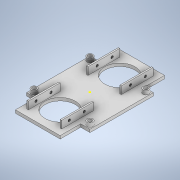
# Autodesk Inventor part: hydra_spider_v4_o
Saved by Autodesk Inventor 2020 (Build 240168000, 168)
## iProperties
Created: 2022-08-29
Part Number: hydra_spider_v4_o
Material: Generic
Document SubType Name: Modeling
Designer: Administrator
Density: 1 g/cm^3
Appearance: Default
Author: Administrator
Autodesk Inventor part; units mm, degrees
ref_plane "YZ Plane" through (0, 0, 0) normal (1, 0, 0) x (0, 1, 0)
ref_plane "XZ Plane" through (0, 0, 0) normal (0, 1, 0) x (-1, 0, 0)
ref_plane "XY Plane" through (0, 0, 0) normal (0, 0, 1) x (1, 0, 0)
sketch "Sketch1" plane through (0, 0, 0) normal (0, 1, 0) x (-1, 0, 0)
  line L0 (-42.5, -42.5) -> (42.5, -42.5)
  line L1 (42.5, -42.5) -> (42.5, 42.5)
  line L2 (42.5, 42.5) -> (-42.5, 42.5)
  line L3 (-42.5, 42.5) -> (-42.5, -42.5)
  line L4 (-45, -45) -> (40, 40) construction
  line L5 (40, -45) -> (-45, 40) construction
  line L6 (37.5, -37.5) -> (37.5, 37.5)
  line L7 (37.5, 37.5) -> (-37.5, 37.5)
  line L8 (-37.5, -37.5) -> (37.5, 37.5) construction
  line L9 (37.5, -37.5) -> (-37.5, 37.5) construction
  circle A0 centre (37.5, 37.5) radius 2.6
  line L10 (-36, -36) -> (36, 36) construction
  line L11 (36, -36) -> (-36, 36) construction
  circle A1 centre (37.5, -37.5) radius 2.6
  circle A2 centre (-37.5, 37.5) radius 2.6
  circle A3 centre (-37.5, -37.5) radius 2.6
  line L12 (30, -40) -> (-30, -40)
  line L13 (-30, -40) -> (-30, -70)
  line L14 (-30, -70) -> (30, -70)
  line L15 (30, -70) -> (30, -40)
  line L16 (-30, -40) -> (-30, 40)
  line L17 (30, 70) -> (-30, 70)
  line L18 (-30, 70) -> (-30, 40)
  line L19 (-30, 40) -> (30, 40)
  line L20 (30, 40) -> (30, 70)
  circle A4 centre (0, -40) radius 20.25
  circle A5 centre (0, 40) radius 20.25
  line L21 (55.4392, 43.942) -> (57.9392, 43.942)
  line L22 (57.9392, 43.942) -> (57.9392, 46.442)
  point P0 (20.0951, 37.5)
  point P1 (-20.0951, 37.5)
  point P2 (-30, 42.5)
  point P3 (-30, -42.5)
  point P4 (30, -42.5)
  point P5 (30, 42.5)
  point P6 (-20.0951, 42.5)
  point P7 (20.0951, 42.5)
  point P8 (37.5, 34.9)
  point P9 (34.9, 37.5)
  dimension "d0" = 85
  dimension "d1" = 85
  dimension "d2" = 75
  dimension "d3" = 75
  dimension "d4" = 5.2
  dimension "d5" = 72
  dimension "d6" = 72
  dimension "d9" = 75
  dimension "d12" = 75
  dimension "d164" = 60
  dimension "d165" = 30
  dimension "d170" = 60
  dimension "d171" = 30
  dimension "d172" = 40.5
  dimension "d173" = 40.5
  dimension "d441" = 2.5
  dimension "d442" = 2.5
  constraints: 46 end point, 6 centre point, 6 parallel, 5 horizontal, 5 perpendicular, 2 midpoint, 1 coincident, 1 vertical, 6 other
  measures "d0" distance of L2.end L1.end
  measures "d1" distance of L1.end L0.end
  measures "d2" distance of L7.end L6.end
  measures "d3" distance of L6.end L6.start
  measures "d4" diameter of A0
  measures "d5" distance of L11.end L10.end
  measures "d6" distance of L10.end L11.start
  measures "d9" distance of A0.centre A1.centre
  measures "d12" distance of A0.centre A2.centre
  measures "d164" distance of L14.end L13.end
  measures "d165" distance of L12.end L13.end
  measures "d170" distance of L20.start L18.end
  measures "d171" distance of L17.end L18.end
  measures "d172" diameter of A4
  measures "d173" diameter of A5
  measures "d441" distance of L21.start L21.end
  measures "d442" distance of L21.end L22.end
extrude "Extrusion1" add sketch "Sketch1" along normal blind 4 contours A2 | L3 L2 L18 L16 L13 L0 | L13 L12 A4 L0 | L0 A4 L15 L14 L13 | A1 | A0 L6 L7 | L7 L6 A0 | L16 L7 A5 L19 L20 L2 L1 L0 L15 L12 A4 | L18 L17 L20 L2 A5 | L2 A5 L19 L18 | A4 L12 L15 L0 | L16 L19 A5 L7 | L2 L20 L19 A5 | A3
sketch "Sketch2" plane through (0, 4, 0) normal (0, 1, 0) x (1, 0, 0)
  line L0 (0, 0) -> (21.3, 0)
  line L1 (21.3, 61.3) -> (21.3, 18.7)
  line L2 (21.3, 61.3) -> (-21.3, 61.3)
  line L3 (-21.3, 61.3) -> (-21.3, 18.7)
  line L4 (-21.3, 18.7) -> (-23.3, 18.7)
  line L5 (-23.3, 18.7) -> (-23.3, 61.3)
  line L6 (23.3, 61.3) -> (23.3, 18.7)
  line L7 (23.3, 18.7) -> (21.3, 18.7)
  line L8 (21.3, -61.3) -> (21.3, -18.7)
  line L9 (-21.3, -61.3) -> (-21.3, -18.7)
  line L10 (-21.3, -18.7) -> (-23.3, -18.7)
  line L11 (-23.3, -18.7) -> (-23.3, -61.3)
  line L12 (23.3, -61.3) -> (23.3, -18.7)
  line L13 (23.3, -18.7) -> (21.3, -18.7)
  line L14 (-23.3, -61.3) -> (-21.3, -61.3)
  line L15 (21.3, -61.3) -> (23.3, -61.3)
  line L16 (-23.3, 61.3) -> (-21.3, 61.3)
  line L17 (21.3, 61.3) -> (23.3, 61.3)
  line L18 (-23.3, 63.3) -> (-21.3, 63.3)
  line L19 (21.3, 63.3) -> (23.3, 63.3)
  dimension "d176" = 42.6
  dimension "d177" = 42.6
  dimension "d178" = 42.6
  dimension "d179" = 2
  dimension "d180" = 44.6
  dimension "d181" = 46.6
  constraints: 40 end point, 10 perpendicular, 6 symmetric about line, 5 point on line, 2 horizontal
  measures "d176" distance of L1.start L1.end
  measures "d177" distance of L1.start L2.end
  measures "d178" distance of L2.end L3.end
  measures "d179" distance of L3.end L4.end
  measures "d180" distance of L4.end L18.start
  measures "d181" distance of L18.start L19.end
extrude "Extrusion2" add sketch "Sketch2" along normal blind 10
sketch "Sketch18" plane through (-23.3, 4, 18.7) normal (-1, 0, 0) x (0, 0, 1)
  line L0 (-80, 10) -> (-37.4, 10) projected
  line L1 (-59.7, 10) -> (-59.7, 0)
  line L2 (-88.7, 0) -> (-61.2, 0) projected
  line L3 (-49.7, 5) -> (-69.7, 5)
  line L4 (42.6, 10) -> (0, 10) projected
  line L5 (22.3, 10) -> (22.3, 0)
  line L6 (51.3, 0) -> (23.8, 0) projected
  circle A0 centre (-49.7, 5) radius 1.65
  circle A1 centre (-69.7, 5) radius 1.65
  line L7 (-59.7, 0) -> (-59.7, 5)
  line L8 (22.3, 0) -> (22.3, 5)
  circle A2 centre (32.3, 5) radius 1.65
  circle A3 centre (12.3, 5) radius 1.65
  point P0 (-18.7, -4)
  point P1 (-82, 10)
  point P2 (44.6, 10)
  dimension "d191" = 20
  dimension "d192" = 3.3
  dimension "d193" = 3.3
  dimension "d194" = 20
  dimension "d195" = 3.3
  dimension "d196" = 3.3
  constraints: 10 end point, 4 centre point, 4 coincident, 4 point on line, 2 midpoint, 2 vertical
  measures "d191" distance of L3.start L3.end
  measures "d192" diameter of A0
  measures "d193" diameter of A1
  measures "d194" distance of point (32.3, 5) point (12.3, 5)
  measures "d195" diameter of A2
  measures "d196" diameter of A3
extrude "Extrusion6" cut sketch "Sketch18" against normal through all
thread "Thread7" size "M3x0.5" class "6H" standard "ANSI Metric M Profile" full length
thread "Thread8" size "M3x0.5" class "6H" standard "ANSI Metric M Profile" full length
thread "Thread11" size "M3x0.5" class "6H" standard "ANSI Metric M Profile" full length
thread "Thread12" size "M3x0.5" class "6H" standard "ANSI Metric M Profile" full length
thread "Thread13" size "M3x0.5" class "6H" standard "ANSI Metric M Profile" full length
thread "Thread14" size "M3x0.5" class "6H" standard "ANSI Metric M Profile" full length
thread "Thread15" size "M3x0.5" class "6H" standard "ANSI Metric M Profile" full length
thread "Thread16" size "M3x0.5" class "6H" standard "ANSI Metric M Profile" full length
sketch "Sketch20" plane through (-21.3, 9, -31) normal (0, -1, 0) x (0, 0, 1)
  line L0 (1.65, 0) -> (1.65, 2)
  line L1 (1.65, 2) -> (1.2793, 2)
  line L2 (1.2793, 2) -> (1.2793, 0)
  line L3 (1.2793, 0) -> (1.65, 0)
  line L4 (0, -25.96) -> (0, 6.66) projected
  constraints: 8 end point
revolve "Revolution7" add sketch "Sketch20" angle 360 about axis through (-21.3, 9, -31) along (-1, 0, 0) separate body
sketch "Sketch19" plane through (-21.3, 9, -29.35) normal (0, 1, 0) x (-1, 0, 0)
  line L0 (-0.2918, -0.0255) -> (-0.2501, -0.0255) construction
  line L1 (0.0416, -0.3456) -> (-0.0001, -0.4257) construction
  line L2 (-0.5001, -0.4257) -> (-0.5418, -0.3456) construction
  line L3 (-0.2084, -0.0255) -> (-0.2501, 0.0546) construction
  line L4 (-0.2501, 0.0546) -> (-0.2918, -0.0255) construction
  line L5 (-0.5001, -0.4257) -> (-0.4584, -0.3456) construction
  line L6 (-0.2084, -0.0255) -> (-0.0418, -0.3456)
  line L7 (-0.5418, -0.3456) -> (-0.4584, -0.3456) construction
  arc A0 (-0.5418, -0.3456) -> (-0.5001, -0.3709) centre (-0.5001, -0.3239) ccw construction
  line L8 (0.0416, -0.3456) -> (-0.0418, -0.3456) construction
  line L9 (-0.5001, -0.4257) -> (-0.5001, -0.3456) construction
  line L10 (-0.0001, -0.4257) -> (-0.0001, -0.3456) construction
  line L11 (-0.2501, 0.0546) -> (-0.2501, -0.0002) construction
  line L12 (-0.5001, -0.3709) -> (-0.0001, -0.3709)
  arc A1 (-0.5001, -0.3709) -> (-0.4584, -0.3456) centre (-0.5001, -0.3239) ccw
  line L13 (-0.0418, -0.3456) -> (-0.0001, -0.4257) construction
  line L14 (-0.4584, -0.3456) -> (-0.2918, -0.0255)
  line L15 (-0.0001, -0.0002) -> (-0.0001, 0.0177)
  line L16 (-0.0001, 0.0177) -> (-0.0001, -0.0002)
  line L17 (-0.0001, -0.0002) -> (0.0334, -0.0002)
  arc A2 (-0.0418, -0.3456) -> (-0.0001, -0.3709) centre (-0.0001, -0.3239) ccw
  arc A3 (-0.0001, -0.3709) -> (0.0416, -0.3456) centre (-0.0001, -0.3239) ccw construction
  arc A4 (-0.2501, -0.0002) -> (-0.2918, -0.0255) centre (-0.2501, -0.0471) ccw
  arc A5 (-0.2084, -0.0255) -> (-0.2501, -0.0002) centre (-0.2501, -0.0471) ccw
  line L18 (-0.2501, -0.0002) -> (-0.2501, -0.0255) construction
  line L19 (-0.2501, -0.0255) -> (-0.2084, -0.0255) construction
  dimension "d225" = 55
  dimension "d226" = 0.08
  dimension "d227" = 0.08
  dimension "Sketch19_ThreadOffset" = 0
  dimension "Sketch19_MajorRadius" = 0.3707
  dimension "d230" = 0.5
  dimension "Sketch19_MinorRadius" = 0
  constraints: 40 end point, 12 point on circle, 10 parallel, 8 tangent, 6 centre point, 6 collinear, 2 midpoint, 2 point on line, 1 horizontal, 1 perpendicular, 3 other
  measures "d225" angle of L6 L14
  measures "d226" distance of L3.end L0.end
  measures "d227" distance of L1.end L10.end
  measures "Sketch19_ThreadOffset" distance between parallel lines of L15 L10
  measures "Sketch19_MajorRadius" distance from line of L12 L15.start
  measures "d230" distance from line of L1.end L9
  measures "Sketch19_MinorRadius" distance edge to line of A5 L17
coil "Coil7" sketch "Sketch19" operation cut axis through (-21.3, 9, -31) along (-1, 0, 0) pitch 0.5005 turns 5.994006 hand right bodies 2
sketch "Sketch22" plane through (-21.3, 9, -51) normal (0, -1, 0) x (0, 0, 1)
  line L0 (1.65, 0) -> (1.65, 2)
  line L1 (1.65, 2) -> (1.2793, 2)
  line L2 (1.2793, 2) -> (1.2793, 0)
  line L3 (1.2793, 0) -> (1.65, 0)
  line L4 (0, -25.96) -> (0, 6.66) projected
  constraints: 8 end point
revolve "Revolution8" add sketch "Sketch22" angle 360 about axis through (-21.3, 9, -51) along (-1, 0, 0) separate body
sketch "Sketch21" plane through (-21.3, 9, -49.35) normal (0, 1, 0) x (-1, 0, 0)
  line L0 (-0.2918, -0.0255) -> (-0.2501, -0.0255) construction
  line L1 (0.0416, -0.3456) -> (-0.0001, -0.4257) construction
  line L2 (-0.5001, -0.4257) -> (-0.5418, -0.3456) construction
  line L3 (-0.2084, -0.0255) -> (-0.2501, 0.0546) construction
  line L4 (-0.2501, 0.0546) -> (-0.2918, -0.0255) construction
  line L5 (-0.5001, -0.4257) -> (-0.4584, -0.3456) construction
  line L6 (-0.2084, -0.0255) -> (-0.0418, -0.3456)
  line L7 (-0.5418, -0.3456) -> (-0.4584, -0.3456) construction
  arc A0 (-0.5418, -0.3456) -> (-0.5001, -0.3709) centre (-0.5001, -0.3239) ccw construction
  line L8 (0.0416, -0.3456) -> (-0.0418, -0.3456) construction
  line L9 (-0.5001, -0.4257) -> (-0.5001, -0.3456) construction
  line L10 (-0.0001, -0.4257) -> (-0.0001, -0.3456) construction
  line L11 (-0.2501, 0.0546) -> (-0.2501, -0.0002) construction
  line L12 (-0.5001, -0.3709) -> (-0.0001, -0.3709)
  arc A1 (-0.5001, -0.3709) -> (-0.4584, -0.3456) centre (-0.5001, -0.3239) ccw
  line L13 (-0.0418, -0.3456) -> (-0.0001, -0.4257) construction
  line L14 (-0.4584, -0.3456) -> (-0.2918, -0.0255)
  line L15 (-0.0001, -0.0002) -> (-0.0001, 0.0177)
  line L16 (-0.0001, 0.0177) -> (-0.0001, -0.0002)
  line L17 (-0.0001, -0.0002) -> (0.0334, -0.0002)
  arc A2 (-0.0418, -0.3456) -> (-0.0001, -0.3709) centre (-0.0001, -0.3239) ccw
  arc A3 (-0.0001, -0.3709) -> (0.0416, -0.3456) centre (-0.0001, -0.3239) ccw construction
  arc A4 (-0.2501, -0.0002) -> (-0.2918, -0.0255) centre (-0.2501, -0.0471) ccw
  arc A5 (-0.2084, -0.0255) -> (-0.2501, -0.0002) centre (-0.2501, -0.0471) ccw
  line L18 (-0.2501, -0.0002) -> (-0.2501, -0.0255) construction
  line L19 (-0.2501, -0.0255) -> (-0.2084, -0.0255) construction
  dimension "d243" = 55
  dimension "d244" = 0.08
  dimension "d245" = 0.08
  dimension "Sketch21_ThreadOffset" = 0
  dimension "Sketch21_MajorRadius" = 0.3707
  dimension "d248" = 0.5
  dimension "Sketch21_MinorRadius" = 0
  constraints: 40 end point, 12 point on circle, 10 parallel, 8 tangent, 6 centre point, 6 collinear, 2 midpoint, 2 point on line, 1 horizontal, 1 perpendicular, 3 other
  measures "d243" angle of L6 L14
  measures "d244" distance of L3.end L0.end
  measures "d245" distance of L1.end L10.end
  measures "Sketch21_ThreadOffset" distance between parallel lines of L15 L10
  measures "Sketch21_MajorRadius" distance from line of L12 L15.start
  measures "d248" distance from line of L1.end L9
  measures "Sketch21_MinorRadius" distance edge to line of A5 L17
coil "Coil8" sketch "Sketch21" operation cut axis through (-21.3, 9, -51) along (-1, 0, 0) pitch 0.5005 turns 5.994006 hand right bodies 3
sketch "Sketch28" plane through (23.3, 9, -51) normal (0, -1, 0) x (0, 0, 1)
  line L0 (1.65, 0) -> (1.65, 2)
  line L1 (1.65, 2) -> (1.2793, 2)
  line L2 (1.2793, 2) -> (1.2793, 0)
  line L3 (1.2793, 0) -> (1.65, 0)
  line L4 (0, -4.66) -> (0, 27.96) projected
  constraints: 8 end point
revolve "Revolution11" add sketch "Sketch28" angle 360 about axis through (23.3, 9, -51) along (-1, 0, 0) separate body
sketch "Sketch27" plane through (23.3, 9, -49.35) normal (0, 1, 0) x (-1, 0, 0)
  line L0 (-0.2918, -0.0255) -> (-0.2501, -0.0255) construction
  line L1 (0.0416, -0.3456) -> (-0.0001, -0.4257) construction
  line L2 (-0.5001, -0.4257) -> (-0.5418, -0.3456) construction
  line L3 (-0.2084, -0.0255) -> (-0.2501, 0.0546) construction
  line L4 (-0.2501, 0.0546) -> (-0.2918, -0.0255) construction
  line L5 (-0.5001, -0.4257) -> (-0.4584, -0.3456) construction
  line L6 (-0.2084, -0.0255) -> (-0.0418, -0.3456)
  line L7 (-0.5418, -0.3456) -> (-0.4584, -0.3456) construction
  arc A0 (-0.5418, -0.3456) -> (-0.5001, -0.3709) centre (-0.5001, -0.3239) ccw construction
  line L8 (0.0416, -0.3456) -> (-0.0418, -0.3456) construction
  line L9 (-0.5001, -0.4257) -> (-0.5001, -0.3456) construction
  line L10 (-0.0001, -0.4257) -> (-0.0001, -0.3456) construction
  line L11 (-0.2501, 0.0546) -> (-0.2501, -0.0002) construction
  line L12 (-0.5001, -0.3709) -> (-0.0001, -0.3709)
  arc A1 (-0.5001, -0.3709) -> (-0.4584, -0.3456) centre (-0.5001, -0.3239) ccw
  line L13 (-0.0418, -0.3456) -> (-0.0001, -0.4257) construction
  line L14 (-0.4584, -0.3456) -> (-0.2918, -0.0255)
  line L15 (-0.0001, -0.0002) -> (-0.0001, 0.0177)
  line L16 (-0.0001, 0.0177) -> (-0.0001, -0.0002)
  line L17 (-0.0001, -0.0002) -> (0.0334, -0.0002)
  arc A2 (-0.0418, -0.3456) -> (-0.0001, -0.3709) centre (-0.0001, -0.3239) ccw
  arc A3 (-0.0001, -0.3709) -> (0.0416, -0.3456) centre (-0.0001, -0.3239) ccw construction
  arc A4 (-0.2501, -0.0002) -> (-0.2918, -0.0255) centre (-0.2501, -0.0471) ccw
  arc A5 (-0.2084, -0.0255) -> (-0.2501, -0.0002) centre (-0.2501, -0.0471) ccw
  line L18 (-0.2501, -0.0002) -> (-0.2501, -0.0255) construction
  line L19 (-0.2501, -0.0255) -> (-0.2084, -0.0255) construction
  dimension "d297" = 55
  dimension "d298" = 0.08
  dimension "d299" = 0.08
  dimension "Sketch27_ThreadOffset" = 0
  dimension "Sketch27_MajorRadius" = 0.3707
  dimension "d302" = 0.5
  dimension "Sketch27_MinorRadius" = 0
  constraints: 40 end point, 12 point on circle, 10 parallel, 8 tangent, 6 centre point, 6 collinear, 2 midpoint, 2 point on line, 1 horizontal, 1 perpendicular, 3 other
  measures "d297" angle of L6 L14
  measures "d298" distance of L3.end L0.end
  measures "d299" distance of L1.end L10.end
  measures "Sketch27_ThreadOffset" distance between parallel lines of L15 L10
  measures "Sketch27_MajorRadius" distance from line of L12 L15.start
  measures "d302" distance from line of L1.end L9
  measures "Sketch27_MinorRadius" distance edge to line of A5 L17
coil "Coil11" sketch "Sketch27" operation cut axis through (23.3, 9, -51) along (-1, 0, 0) pitch 0.5005 turns 5.994006 hand right bodies 4
sketch "Sketch30" plane through (23.3, 9, -31) normal (0, -1, 0) x (0, 0, 1)
  line L0 (1.65, 0) -> (1.65, 2)
  line L1 (1.65, 2) -> (1.2793, 2)
  line L2 (1.2793, 2) -> (1.2793, 0)
  line L3 (1.2793, 0) -> (1.65, 0)
  line L4 (0, -4.66) -> (0, 27.96) projected
  constraints: 8 end point
revolve "Revolution12" add sketch "Sketch30" angle 360 about axis through (23.3, 9, -31) along (-1, 0, 0) separate body
sketch "Sketch29" plane through (23.3, 9, -29.35) normal (0, 1, 0) x (-1, 0, 0)
  line L0 (-0.2918, -0.0255) -> (-0.2501, -0.0255) construction
  line L1 (0.0416, -0.3456) -> (-0.0001, -0.4257) construction
  line L2 (-0.5001, -0.4257) -> (-0.5418, -0.3456) construction
  line L3 (-0.2084, -0.0255) -> (-0.2501, 0.0546) construction
  line L4 (-0.2501, 0.0546) -> (-0.2918, -0.0255) construction
  line L5 (-0.5001, -0.4257) -> (-0.4584, -0.3456) construction
  line L6 (-0.2084, -0.0255) -> (-0.0418, -0.3456)
  line L7 (-0.5418, -0.3456) -> (-0.4584, -0.3456) construction
  arc A0 (-0.5418, -0.3456) -> (-0.5001, -0.3709) centre (-0.5001, -0.3239) ccw construction
  line L8 (0.0416, -0.3456) -> (-0.0418, -0.3456) construction
  line L9 (-0.5001, -0.4257) -> (-0.5001, -0.3456) construction
  line L10 (-0.0001, -0.4257) -> (-0.0001, -0.3456) construction
  line L11 (-0.2501, 0.0546) -> (-0.2501, -0.0002) construction
  line L12 (-0.5001, -0.3709) -> (-0.0001, -0.3709)
  arc A1 (-0.5001, -0.3709) -> (-0.4584, -0.3456) centre (-0.5001, -0.3239) ccw
  line L13 (-0.0418, -0.3456) -> (-0.0001, -0.4257) construction
  line L14 (-0.4584, -0.3456) -> (-0.2918, -0.0255)
  line L15 (-0.0001, -0.0002) -> (-0.0001, 0.0177)
  line L16 (-0.0001, 0.0177) -> (-0.0001, -0.0002)
  line L17 (-0.0001, -0.0002) -> (0.0334, -0.0002)
  arc A2 (-0.0418, -0.3456) -> (-0.0001, -0.3709) centre (-0.0001, -0.3239) ccw
  arc A3 (-0.0001, -0.3709) -> (0.0416, -0.3456) centre (-0.0001, -0.3239) ccw construction
  arc A4 (-0.2501, -0.0002) -> (-0.2918, -0.0255) centre (-0.2501, -0.0471) ccw
  arc A5 (-0.2084, -0.0255) -> (-0.2501, -0.0002) centre (-0.2501, -0.0471) ccw
  line L18 (-0.2501, -0.0002) -> (-0.2501, -0.0255) construction
  line L19 (-0.2501, -0.0255) -> (-0.2084, -0.0255) construction
  dimension "d315" = 55
  dimension "d316" = 0.08
  dimension "d317" = 0.08
  dimension "Sketch29_ThreadOffset" = 0
  dimension "Sketch29_MajorRadius" = 0.3707
  dimension "d320" = 0.5
  dimension "Sketch29_MinorRadius" = 0
  constraints: 40 end point, 12 point on circle, 10 parallel, 8 tangent, 6 centre point, 6 collinear, 2 midpoint, 2 point on line, 1 horizontal, 1 perpendicular, 3 other
  measures "d315" angle of L6 L14
  measures "d316" distance of L3.end L0.end
  measures "d317" distance of L1.end L10.end
  measures "Sketch29_ThreadOffset" distance between parallel lines of L15 L10
  measures "Sketch29_MajorRadius" distance from line of L12 L15.start
  measures "d320" distance from line of L1.end L9
  measures "Sketch29_MinorRadius" distance edge to line of A5 L17
coil "Coil12" sketch "Sketch29" operation cut axis through (23.3, 9, -31) along (-1, 0, 0) pitch 0.5005 turns 5.994006 hand right bodies 5
sketch "Sketch32" plane through (23.3, 9, 31) normal (0, -1, 0) x (0, 0, 1)
  line L0 (1.65, 0) -> (1.65, 2)
  line L1 (1.65, 2) -> (1.2793, 2)
  line L2 (1.2793, 2) -> (1.2793, 0)
  line L3 (1.2793, 0) -> (1.65, 0)
  line L4 (0, -4.66) -> (0, 27.96) projected
  constraints: 8 end point
revolve "Revolution13" add sketch "Sketch32" angle 360 about axis through (23.3, 9, 31) along (-1, 0, 0) separate body
sketch "Sketch31" plane through (23.3, 9, 32.65) normal (0, 1, 0) x (-1, 0, 0)
  line L0 (-0.2918, -0.0255) -> (-0.2501, -0.0255) construction
  line L1 (0.0416, -0.3456) -> (-0.0001, -0.4257) construction
  line L2 (-0.5001, -0.4257) -> (-0.5418, -0.3456) construction
  line L3 (-0.2084, -0.0255) -> (-0.2501, 0.0546) construction
  line L4 (-0.2501, 0.0546) -> (-0.2918, -0.0255) construction
  line L5 (-0.5001, -0.4257) -> (-0.4584, -0.3456) construction
  line L6 (-0.2084, -0.0255) -> (-0.0418, -0.3456)
  line L7 (-0.5418, -0.3456) -> (-0.4584, -0.3456) construction
  arc A0 (-0.5418, -0.3456) -> (-0.5001, -0.3709) centre (-0.5001, -0.3239) ccw construction
  line L8 (0.0416, -0.3456) -> (-0.0418, -0.3456) construction
  line L9 (-0.5001, -0.4257) -> (-0.5001, -0.3456) construction
  line L10 (-0.0001, -0.4257) -> (-0.0001, -0.3456) construction
  line L11 (-0.2501, 0.0546) -> (-0.2501, -0.0002) construction
  line L12 (-0.5001, -0.3709) -> (-0.0001, -0.3709)
  arc A1 (-0.5001, -0.3709) -> (-0.4584, -0.3456) centre (-0.5001, -0.3239) ccw
  line L13 (-0.0418, -0.3456) -> (-0.0001, -0.4257) construction
  line L14 (-0.4584, -0.3456) -> (-0.2918, -0.0255)
  line L15 (-0.0001, -0.0002) -> (-0.0001, 0.0177)
  line L16 (-0.0001, 0.0177) -> (-0.0001, -0.0002)
  line L17 (-0.0001, -0.0002) -> (0.0334, -0.0002)
  arc A2 (-0.0418, -0.3456) -> (-0.0001, -0.3709) centre (-0.0001, -0.3239) ccw
  arc A3 (-0.0001, -0.3709) -> (0.0416, -0.3456) centre (-0.0001, -0.3239) ccw construction
  arc A4 (-0.2501, -0.0002) -> (-0.2918, -0.0255) centre (-0.2501, -0.0471) ccw
  arc A5 (-0.2084, -0.0255) -> (-0.2501, -0.0002) centre (-0.2501, -0.0471) ccw
  line L18 (-0.2501, -0.0002) -> (-0.2501, -0.0255) construction
  line L19 (-0.2501, -0.0255) -> (-0.2084, -0.0255) construction
  dimension "d333" = 55
  dimension "d334" = 0.08
  dimension "d335" = 0.08
  dimension "Sketch31_ThreadOffset" = 0
  dimension "Sketch31_MajorRadius" = 0.3707
  dimension "d338" = 0.5
  dimension "Sketch31_MinorRadius" = 0
  constraints: 40 end point, 12 point on circle, 10 parallel, 8 tangent, 6 centre point, 6 collinear, 2 midpoint, 2 point on line, 1 horizontal, 1 perpendicular, 3 other
  measures "d333" angle of L6 L14
  measures "d334" distance of L3.end L0.end
  measures "d335" distance of L1.end L10.end
  measures "Sketch31_ThreadOffset" distance between parallel lines of L15 L10
  measures "Sketch31_MajorRadius" distance from line of L12 L15.start
  measures "d338" distance from line of L1.end L9
  measures "Sketch31_MinorRadius" distance edge to line of A5 L17
coil "Coil13" sketch "Sketch31" operation cut axis through (23.3, 9, 31) along (-1, 0, 0) pitch 0.5005 turns 5.994006 hand right bodies 6
sketch "Sketch34" plane through (23.3, 9, 51) normal (0, -1, 0) x (0, 0, 1)
  line L0 (1.65, 0) -> (1.65, 2)
  line L1 (1.65, 2) -> (1.2793, 2)
  line L2 (1.2793, 2) -> (1.2793, 0)
  line L3 (1.2793, 0) -> (1.65, 0)
  line L4 (0, -4.66) -> (0, 27.96) projected
  constraints: 8 end point
revolve "Revolution14" add sketch "Sketch34" angle 360 about axis through (23.3, 9, 51) along (-1, 0, 0) separate body
sketch "Sketch33" plane through (23.3, 9, 52.65) normal (0, 1, 0) x (-1, 0, 0)
  line L0 (-0.2918, -0.0255) -> (-0.2501, -0.0255) construction
  line L1 (0.0416, -0.3456) -> (-0.0001, -0.4257) construction
  line L2 (-0.5001, -0.4257) -> (-0.5418, -0.3456) construction
  line L3 (-0.2084, -0.0255) -> (-0.2501, 0.0546) construction
  line L4 (-0.2501, 0.0546) -> (-0.2918, -0.0255) construction
  line L5 (-0.5001, -0.4257) -> (-0.4584, -0.3456) construction
  line L6 (-0.2084, -0.0255) -> (-0.0418, -0.3456)
  line L7 (-0.5418, -0.3456) -> (-0.4584, -0.3456) construction
  arc A0 (-0.5418, -0.3456) -> (-0.5001, -0.3709) centre (-0.5001, -0.3239) ccw construction
  line L8 (0.0416, -0.3456) -> (-0.0418, -0.3456) construction
  line L9 (-0.5001, -0.4257) -> (-0.5001, -0.3456) construction
  line L10 (-0.0001, -0.4257) -> (-0.0001, -0.3456) construction
  line L11 (-0.2501, 0.0546) -> (-0.2501, -0.0002) construction
  line L12 (-0.5001, -0.3709) -> (-0.0001, -0.3709)
  arc A1 (-0.5001, -0.3709) -> (-0.4584, -0.3456) centre (-0.5001, -0.3239) ccw
  line L13 (-0.0418, -0.3456) -> (-0.0001, -0.4257) construction
  line L14 (-0.4584, -0.3456) -> (-0.2918, -0.0255)
  line L15 (-0.0001, -0.0002) -> (-0.0001, 0.0177)
  line L16 (-0.0001, 0.0177) -> (-0.0001, -0.0002)
  line L17 (-0.0001, -0.0002) -> (0.0334, -0.0002)
  arc A2 (-0.0418, -0.3456) -> (-0.0001, -0.3709) centre (-0.0001, -0.3239) ccw
  arc A3 (-0.0001, -0.3709) -> (0.0416, -0.3456) centre (-0.0001, -0.3239) ccw construction
  arc A4 (-0.2501, -0.0002) -> (-0.2918, -0.0255) centre (-0.2501, -0.0471) ccw
  arc A5 (-0.2084, -0.0255) -> (-0.2501, -0.0002) centre (-0.2501, -0.0471) ccw
  line L18 (-0.2501, -0.0002) -> (-0.2501, -0.0255) construction
  line L19 (-0.2501, -0.0255) -> (-0.2084, -0.0255) construction
  dimension "d351" = 55
  dimension "d352" = 0.08
  dimension "d353" = 0.08
  dimension "Sketch33_ThreadOffset" = 0
  dimension "Sketch33_MajorRadius" = 0.3707
  dimension "d356" = 0.5
  dimension "Sketch33_MinorRadius" = 0
  constraints: 40 end point, 12 point on circle, 10 parallel, 8 tangent, 6 centre point, 6 collinear, 2 midpoint, 2 point on line, 1 horizontal, 1 perpendicular, 3 other
  measures "d351" angle of L6 L14
  measures "d352" distance of L3.end L0.end
  measures "d353" distance of L1.end L10.end
  measures "Sketch33_ThreadOffset" distance between parallel lines of L15 L10
  measures "Sketch33_MajorRadius" distance from line of L12 L15.start
  measures "d356" distance from line of L1.end L9
  measures "Sketch33_MinorRadius" distance edge to line of A5 L17
coil "Coil14" sketch "Sketch33" operation cut axis through (23.3, 9, 51) along (-1, 0, 0) pitch 0.5005 turns 5.994006 hand right bodies 7
sketch "Sketch36" plane through (-21.3, 9, 31) normal (0, -1, 0) x (0, 0, 1)
  line L0 (1.65, 0) -> (1.65, 2)
  line L1 (1.65, 2) -> (1.2793, 2)
  line L2 (1.2793, 2) -> (1.2793, 0)
  line L3 (1.2793, 0) -> (1.65, 0)
  line L4 (0, -25.96) -> (0, 6.66) projected
  constraints: 8 end point
revolve "Revolution15" add sketch "Sketch36" angle 360 about axis through (-21.3, 9, 31) along (-1, 0, 0) separate body
sketch "Sketch35" plane through (-21.3, 9, 32.65) normal (0, 1, 0) x (-1, 0, 0)
  line L0 (-0.2918, -0.0255) -> (-0.2501, -0.0255) construction
  line L1 (0.0416, -0.3456) -> (-0.0001, -0.4257) construction
  line L2 (-0.5001, -0.4257) -> (-0.5418, -0.3456) construction
  line L3 (-0.2084, -0.0255) -> (-0.2501, 0.0546) construction
  line L4 (-0.2501, 0.0546) -> (-0.2918, -0.0255) construction
  line L5 (-0.5001, -0.4257) -> (-0.4584, -0.3456) construction
  line L6 (-0.2084, -0.0255) -> (-0.0418, -0.3456)
  line L7 (-0.5418, -0.3456) -> (-0.4584, -0.3456) construction
  arc A0 (-0.5418, -0.3456) -> (-0.5001, -0.3709) centre (-0.5001, -0.3239) ccw construction
  line L8 (0.0416, -0.3456) -> (-0.0418, -0.3456) construction
  line L9 (-0.5001, -0.4257) -> (-0.5001, -0.3456) construction
  line L10 (-0.0001, -0.4257) -> (-0.0001, -0.3456) construction
  line L11 (-0.2501, 0.0546) -> (-0.2501, -0.0002) construction
  line L12 (-0.5001, -0.3709) -> (-0.0001, -0.3709)
  arc A1 (-0.5001, -0.3709) -> (-0.4584, -0.3456) centre (-0.5001, -0.3239) ccw
  line L13 (-0.0418, -0.3456) -> (-0.0001, -0.4257) construction
  line L14 (-0.4584, -0.3456) -> (-0.2918, -0.0255)
  line L15 (-0.0001, -0.0002) -> (-0.0001, 0.0177)
  line L16 (-0.0001, 0.0177) -> (-0.0001, -0.0002)
  line L17 (-0.0001, -0.0002) -> (0.0334, -0.0002)
  arc A2 (-0.0418, -0.3456) -> (-0.0001, -0.3709) centre (-0.0001, -0.3239) ccw
  arc A3 (-0.0001, -0.3709) -> (0.0416, -0.3456) centre (-0.0001, -0.3239) ccw construction
  arc A4 (-0.2501, -0.0002) -> (-0.2918, -0.0255) centre (-0.2501, -0.0471) ccw
  arc A5 (-0.2084, -0.0255) -> (-0.2501, -0.0002) centre (-0.2501, -0.0471) ccw
  line L18 (-0.2501, -0.0002) -> (-0.2501, -0.0255) construction
  line L19 (-0.2501, -0.0255) -> (-0.2084, -0.0255) construction
  dimension "d369" = 55
  dimension "d370" = 0.08
  dimension "d371" = 0.08
  dimension "Sketch35_ThreadOffset" = 0
  dimension "Sketch35_MajorRadius" = 0.3707
  dimension "d374" = 0.5
  dimension "Sketch35_MinorRadius" = 0
  constraints: 40 end point, 12 point on circle, 10 parallel, 8 tangent, 6 centre point, 6 collinear, 2 midpoint, 2 point on line, 1 horizontal, 1 perpendicular, 3 other
  measures "d369" angle of L6 L14
  measures "d370" distance of L3.end L0.end
  measures "d371" distance of L1.end L10.end
  measures "Sketch35_ThreadOffset" distance between parallel lines of L15 L10
  measures "Sketch35_MajorRadius" distance from line of L12 L15.start
  measures "d374" distance from line of L1.end L9
  measures "Sketch35_MinorRadius" distance edge to line of A5 L17
coil "Coil15" sketch "Sketch35" operation cut axis through (-21.3, 9, 31) along (-1, 0, 0) pitch 0.5005 turns 5.994006 hand right bodies 8
sketch "Sketch38" plane through (-21.3, 9, 51) normal (0, -1, 0) x (0, 0, 1)
  line L0 (1.65, 0) -> (1.65, 2)
  line L1 (1.65, 2) -> (1.2793, 2)
  line L2 (1.2793, 2) -> (1.2793, 0)
  line L3 (1.2793, 0) -> (1.65, 0)
  line L4 (0, -25.96) -> (0, 6.66) projected
  constraints: 8 end point
revolve "Revolution16" add sketch "Sketch38" angle 360 about axis through (-21.3, 9, 51) along (-1, 0, 0) separate body
sketch "Sketch37" plane through (-21.3, 9, 52.65) normal (0, 1, 0) x (-1, 0, 0)
  line L0 (-0.2918, -0.0255) -> (-0.2501, -0.0255) construction
  line L1 (0.0416, -0.3456) -> (-0.0001, -0.4257) construction
  line L2 (-0.5001, -0.4257) -> (-0.5418, -0.3456) construction
  line L3 (-0.2084, -0.0255) -> (-0.2501, 0.0546) construction
  line L4 (-0.2501, 0.0546) -> (-0.2918, -0.0255) construction
  line L5 (-0.5001, -0.4257) -> (-0.4584, -0.3456) construction
  line L6 (-0.2084, -0.0255) -> (-0.0418, -0.3456)
  line L7 (-0.5418, -0.3456) -> (-0.4584, -0.3456) construction
  arc A0 (-0.5418, -0.3456) -> (-0.5001, -0.3709) centre (-0.5001, -0.3239) ccw construction
  line L8 (0.0416, -0.3456) -> (-0.0418, -0.3456) construction
  line L9 (-0.5001, -0.4257) -> (-0.5001, -0.3456) construction
  line L10 (-0.0001, -0.4257) -> (-0.0001, -0.3456) construction
  line L11 (-0.2501, 0.0546) -> (-0.2501, -0.0002) construction
  line L12 (-0.5001, -0.3709) -> (-0.0001, -0.3709)
  arc A1 (-0.5001, -0.3709) -> (-0.4584, -0.3456) centre (-0.5001, -0.3239) ccw
  line L13 (-0.0418, -0.3456) -> (-0.0001, -0.4257) construction
  line L14 (-0.4584, -0.3456) -> (-0.2918, -0.0255)
  line L15 (-0.0001, -0.0002) -> (-0.0001, 0.0177)
  line L16 (-0.0001, 0.0177) -> (-0.0001, -0.0002)
  line L17 (-0.0001, -0.0002) -> (0.0334, -0.0002)
  arc A2 (-0.0418, -0.3456) -> (-0.0001, -0.3709) centre (-0.0001, -0.3239) ccw
  arc A3 (-0.0001, -0.3709) -> (0.0416, -0.3456) centre (-0.0001, -0.3239) ccw construction
  arc A4 (-0.2501, -0.0002) -> (-0.2918, -0.0255) centre (-0.2501, -0.0471) ccw
  arc A5 (-0.2084, -0.0255) -> (-0.2501, -0.0002) centre (-0.2501, -0.0471) ccw
  line L18 (-0.2501, -0.0002) -> (-0.2501, -0.0255) construction
  line L19 (-0.2501, -0.0255) -> (-0.2084, -0.0255) construction
  dimension "d387" = 55
  dimension "d388" = 0.08
  dimension "d389" = 0.08
  dimension "Sketch37_ThreadOffset" = 0
  dimension "Sketch37_MajorRadius" = 0.3707
  dimension "d392" = 0.5
  dimension "Sketch37_MinorRadius" = 0
  constraints: 40 end point, 12 point on circle, 10 parallel, 8 tangent, 6 centre point, 6 collinear, 2 midpoint, 2 point on line, 1 horizontal, 1 perpendicular, 3 other
  measures "d387" angle of L6 L14
  measures "d388" distance of L3.end L0.end
  measures "d389" distance of L1.end L10.end
  measures "Sketch37_ThreadOffset" distance between parallel lines of L15 L10
  measures "Sketch37_MajorRadius" distance from line of L12 L15.start
  measures "d392" distance from line of L1.end L9
  measures "Sketch37_MinorRadius" distance edge to line of A5 L17
coil "Coil16" sketch "Sketch37" operation cut axis through (-21.3, 9, 51) along (-1, 0, 0) pitch 0.5005 turns 5.994006 hand right bodies 9
sketch "Sketch43" plane through (0, 4, 0) normal (0, 1, 0) x (1, 0, 0)
  point P0 (0, 0)
sketch "Sketch44" plane through (0, 4, 0) normal (0, 1, 0) x (1, 0, 0)
  point P0 (0, 0)
sketch "Sketch45" plane through (0, 4, 0) normal (0, 1, 0) x (1, 0, 0)
  line L0 (37.5, 37.5) -> (-37.5, 37.5)
  line L1 (-37.5, 37.5) -> (-37.5, -37.5)
  line L2 (-37.5, -37.5) -> (37.5, -37.5)
  line L3 (37.5, -37.5) -> (37.5, 37.5)
  line L4 (37.5, 37.5) -> (-37.5, -37.5) construction
  line L5 (-37.5, 37.5) -> (37.5, -37.5) construction
  circle A0 centre (37.5, -37.5) radius 2.6
  circle A1 centre (-37.5, -37.5) radius 2.6
  circle A2 centre (37.5, 37.5) radius 2.6
  circle A3 centre (-37.5, 37.5) radius 2.6
  point P0 (0, 0)
  dimension "d443" = 75
  dimension "d444" = 75
  dimension "d445" = 5.2
  dimension "d448" = 75
  dimension "d451" = 75
  constraints: 12 end point, 4 centre point, 2 horizontal, 2 midpoint, 2 parallel, 1 coincident, 1 perpendicular, 1 vertical, 6 other
  measures "d443" distance of L2.end L1.end
  measures "d444" distance of L1.end L0.end
  measures "d445" diameter of A0
  measures "d448" distance of A0.centre A1.centre
  measures "d451" distance of A0.centre A2.centre
extrude "Extrusion7" cut sketch "Sketch45" against normal blind 2 contours A3 L1 L0 | L0 L1 A3 | A2 L3 L0 | L0 L3 A2 | A1 L2 L1 | L1 L2 A1 | A0 L2 L3 | L3 L2 A0 bodies 1
sketch "Sketch46" plane through (0, 4, 0) normal (0, 1, 0) x (1, 0, 0)
  circle A0 centre (37.5, -37.5) radius 2.6 projected
  circle A1 centre (37.5, -37.5) radius 2.6
  circle A2 centre (37.5, -37.5) radius 4
  line L0 (37.5, 37.5) -> (-37.5, 37.5)
  line L1 (-37.5, 37.5) -> (-37.5, -37.5)
  line L2 (-37.5, -37.5) -> (37.5, -37.5)
  line L3 (37.5, -37.5) -> (37.5, 37.5)
  line L4 (37.5, 37.5) -> (-37.5, -37.5) construction
  line L5 (-37.5, 37.5) -> (37.5, -37.5) construction
  circle A3 centre (-37.5, -37.5) radius 2.6
  circle A4 centre (-37.5, -37.5) radius 4
  circle A5 centre (37.5, 37.5) radius 2.6
  circle A6 centre (37.5, 37.5) radius 4
  circle A7 centre (-37.5, 37.5) radius 2.6
  circle A8 centre (-37.5, 37.5) radius 4
  point P0 (0, 0)
  dimension "d456" = 8
  dimension "d457" = 75
  dimension "d458" = 75
  dimension "d461" = 75
  dimension "d464" = 75
  constraints: 12 end point, 8 centre point, 8 coincident, 2 horizontal, 2 midpoint, 2 parallel, 1 perpendicular, 1 vertical, 18 other
  measures "d456" diameter of A2
  measures "d457" distance of L2.end L1.end
  measures "d458" distance of L1.end L0.end
  measures "d461" distance of A1.centre A3.centre
  measures "d464" distance of A1.centre A5.centre
extrude "Extrusion8" add sketch "Sketch46" along normal blind 5 contours A0 L3 A2 L2 | A0 L2 A2 L3 | A6 L0 A5 L3 | L3 A5 L0 A6 | A4 L1 A3 L2 | L2 A3 L1 A4 | A8 L1 A7 L0 | L0 A7 L1 A8 bodies 1
equation "\"d63\" = 55deg"
equation "\"Sketch5_Pitch\" = 0.5"
equation "\"d81\" = 55deg"
equation "\"Sketch7_Pitch\" = 0.5"
equation "\"d99\" = 55deg"
equation "\"Sketch9_Pitch\" = 0.5"
equation "\"d117\" = 55deg"
equation "\"Sketch11_Pitch\" = 0.5"
equation "\"d135\" = 55deg"
equation "\"Sketch13_Pitch\" = 0.5"
equation "\"d153\" = 55deg"
equation "\"Sketch15_Pitch\" = 0.5"
equation "\"d232\" = 55deg"
equation "\"Sketch19_Pitch\" = 0.5"
equation "\"d250\" = 55deg"
equation "\"Sketch21_Pitch\" = 0.5"
equation "\"d268\" = 55deg"
equation "\"Sketch23_Pitch\" = 0.5"
equation "\"d286\" = 55deg"
equation "\"Sketch25_Pitch\" = 0.5"
equation "\"d304\" = 55deg"
equation "\"Sketch27_Pitch\" = 0.5"
equation "\"d322\" = 55deg"
equation "\"Sketch29_Pitch\" = 0.5"
equation "\"d340\" = 55deg"
equation "\"Sketch31_Pitch\" = 0.5"
equation "\"d358\" = 55deg"
equation "\"Sketch33_Pitch\" = 0.5"
equation "\"d376\" = 55deg"
equation "\"Sketch35_Pitch\" = 0.5"
equation "\"d394\" = 55deg"
equation "\"Sketch37_Pitch\" = 0.5"
equation "\"d412\" = 55deg"
equation "\"Sketch39_Pitch\" = 0.5"
equation "\"d430\" = 55deg"
equation "\"Sketch41_Pitch\" = 0.5"
body "Solid1"
body "Solid8"
body "Solid9"
body "Solid12"
body "Solid13"
body "Solid14"
body "Solid15"
body "Solid16"
body "Solid17"
